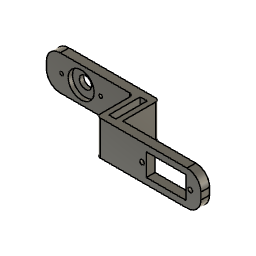
arm_2 v3 (Autodesk Fusion 360 design; units mm, degrees)
Autodesk Fusion 360 part; units mm, degrees
sketch "스케치1" plane through (0, 0, 0) normal (0, 0, 1) x (1, 0, 0)
sketch "스케치2" plane through (0, 0, 0) normal (0, 0, 1) x (1, 0, 0)
sketch "스케치3" plane through (0, 0, 0) normal (0, 0, 1) x (1, 0, 0)
sketch "스케치4" plane through (0, 0, 0) normal (0, 0, 1) x (1, 0, 0)
  line L0 (10, 5) -> (50, 5)
  line L1 (50, 5) -> (50, 0)
  line L2 (50, 0) -> (-20, 0)
  line L3 (-20, 0) -> (-20, 5)
  line L4 (10, 5) -> (10, 22)
  line L5 (10, 22) -> (-20, 22)
  line L6 (-20, 17) -> (-20, 5)
  line L7 (-20, 22) -> (-60, 22)
  line L8 (-60, 22) -> (-60, 17)
  line L9 (-60, 17) -> (-20, 17)
  constraint horizontal L0
  constraint vertical L1
  constraint horizontal L2
  constraint vertical L3
  constraint vertical L4
  constraint horizontal L5
  constraint vertical L6
  constraint horizontal L7
  constraint vertical L8
  constraint horizontal L9
extrude "돌출1" add sketch "스케치4" along normal blind 30
sketch "스케치5" plane through (0, 17, 0) normal (0, -1, 0) x (1, 0, 0)
  circle A0 centre (-40, 15) radius 3.5
  dimension "d3" = 7
  measures "d3" diameter of A0
hole "구멍1" at (-40, 17, 15) direction (0, 1, 0) diameter 7 depth 7 tip angle 118
sketch "스케치6" plane through (0, 17, 0) normal (0, -1, 0) x (1, 0, 0)
  circle A0 centre (-40, 15) radius 7.5
  dimension "d7" = 15
  measures "d7" diameter of A0
extrude "돌출2" cut sketch "스케치6" against normal blind 2.5
sketch "스케치7" plane through (0, 17, 0) normal (0, -1, 0) x (1, 0, 0)
  circle A0 centre (-51.25, 15) radius 1
  dimension "d10" = 2
  measures "d10" diameter of A0
hole "구멍2" at (-51.25, 17, 15) direction (0, 1, 0) diameter 2 depth 7 tip angle 118
sketch "스케치8" plane through (0, 17, 0) normal (0, -1, 0) x (1, 0, 0)
  circle A0 centre (-28.75, 15) radius 1
  dimension "d14" = 2
  measures "d14" diameter of A0
hole "구멍3" at (-28.75, 17, 15) direction (0, 1, 0) diameter 2 depth 7 tip angle 118
sketch "스케치9" plane through (0, 22, 0) normal (0, 1, 0) x (-1, 0, 0)
  circle A0 centre (51.25, 15) radius 1
  circle A1 centre (51.25, 15) radius 3.5
  circle A2 centre (28.75, 15) radius 1
  circle A3 centre (28.75, 15) radius 3.5
  dimension "d18" = 2
  dimension "d19" = 7
  dimension "d20" = 2
  dimension "d21" = 7
  constraint concentric A0 A1
  constraint concentric A2 A3
  measures "d18" diameter of A0
  measures "d19" diameter of A1
  measures "d20" diameter of A2
  measures "d21" diameter of A3
extrude "돌출3" cut sketch "스케치9" against normal blind 1 contours A1
sketch "스케치10" plane through (0, 22, 0) normal (0, 1, 0) x (-1, 0, 0)
  circle A0 centre (28.75, 15) radius 1
  circle A1 centre (28.75, 15) radius 3.5
  dimension "d24" = 2
  dimension "d25" = 7
  constraint concentric A0 A1
  measures "d24" diameter of A0
  measures "d25" diameter of A1
extrude "돌출4" cut sketch "스케치10" against normal blind 1
sketch "스케치11" plane through (0, 5, 0) normal (0, 1, 0) x (-1, 0, 0)
  line L0 (-18.6, 8.6) -> (-41.4, 8.6)
  line L1 (-41.4, 8.6) -> (-41.4, 21.4)
  line L2 (-41.4, 21.4) -> (-18.6, 21.4)
  line L3 (-18.6, 21.4) -> (-18.6, 8.6)
  line L4 (-18.6, 8.6) -> (-41.4, 21.4) construction
  line L5 (-41.4, 8.6) -> (-18.6, 21.4) construction
  point P0 (-30, 15)
  dimension "d28" = 22.8
  dimension "d29" = 12.8
  constraint horizontal L0
  constraint perpendicular L0 L1
  constraint parallel L0 L2
  constraint parallel L1 L3
  constraint coincident L4 P0
  constraint coincident L5 P0
  measures "d28" distance of L1.end L2.end
  measures "d29" distance of L0.end L1.end
extrude "돌출5" cut sketch "스케치11" against normal blind 5
sketch "스케치12" plane through (0, 5, 0) normal (0, 1, 0) x (-1, 0, 0)
  circle A0 centre (-43.9, 15) radius 1.3
  dimension "d32" = 2.6
  measures "d32" diameter of A0
extrude "돌출6" cut sketch "스케치12" against normal blind 5
sketch "스케치13" plane through (0, 5, 0) normal (0, 1, 0) x (-1, 0, 0)
  circle A0 centre (-16.1, 15) radius 1.3
  dimension "d35" = 2.6
  measures "d35" diameter of A0
extrude "돌출7" cut sketch "스케치13" against normal blind 5
extrude "돌출9" cut 1 faces at (-10, 7.3333, 30) along direction (0, 0, -1) blind 5
extrude "돌출10" cut 1 faces at (-10, 7.3333, 0) along direction (0, 0, 1) blind 5
extrude "돌출11" cut 1 faces at (10, 10.6667, 11.6667) along direction (-1, 0, 0) blind 10
extrude "돌출12" cut 1 faces at (-20, 5.6667, 11.6667) along direction (1, 0, 0) blind 10
move_face "면 이동1" to x (1, 0, 0) y (0, 1, 0) z (0, 0, 1) at (0, 4, 0) 12 faces at (-39.6515, 20.3333, 11.5174) (-31.4027, 21, 14.8012) (-28.6504, 18.3333, 14.005) (-53.9027, 21, 14.8012) (-15.9176, 17, 14.9751) (-33.8645, 19.5, 14.5402) (-51.7714, 18.3333, 15.8533) (-54.7326, 21.6667, 14.6515) (-60, 20.3333, 18.3333) (-8.4167, 22, 15) (-32.5093, 18.6667, 14.6262) (-32.2326, 21.6667, 14.6515)
fillet "모깎기18" radius 8 1 edges at (-60, 23.5, 25)
fillet "모깎기19" radius 2 1 edges at (-10, 21, 15)
fillet "모깎기20" radius 2 1 edges at (-10, 0, 15)
fillet "모깎기21" radius 8 1 edges at (-60, 23.5, 5)
fillet "모깎기22" radius 8 1 edges at (50, 2.5, 25)
fillet "모깎기23" radius 8 1 edges at (50, 2.5, 5)
fillet "모깎기24" radius 2 1 edges at (0, 26, 15)
sketch "스케치16" plane through (0, 0, 25) normal (0, 0, 1) x (-1, 0, 0)
  line L0 (7, -22) -> (3, -22)
  line L1 (3, -22) -> (3, -4)
  line L2 (3, -4) -> (7, -4)
  line L3 (7, -4) -> (7, -22)
  constraint horizontal L0
  constraint vertical L1
  constraint horizontal L2
  constraint vertical L3
extrude "돌출13" cut sketch "스케치16" against normal blind 20
sketch "스케치17" plane through (0, 26, 0) normal (0, 1, 0) x (-1, 0, 0)
fillet "모깎기10" [suppressed]
fillet "모깎기11" [suppressed]
fillet "모깎기12" [suppressed]
fillet "모깎기13" [suppressed]
fillet "모깎기14" [suppressed]
fillet "모깎기15" [suppressed]
fillet "모깎기16" [suppressed]
fillet "모깎기17" [suppressed]
sketch "스케치15" plane through (0, 0, 5) normal (0, 0, -1) x (1, 0, 0)
  line L0 (-7, -17) -> (-3, -17)
  line L1 (-3, -17) -> (-3, -3)
  line L2 (-3, -3) -> (-7, -3)
  line L3 (-7, -3) -> (-7, -17)
  line L4 (-7, -17) -> (-3, -3) construction
  line L5 (-3, -17) -> (-7, -3) construction
  point P0 (-5, -10)
  constraint horizontal L0
  constraint perpendicular L0 L1
  constraint parallel L0 L2
  constraint parallel L1 L3
  constraint coincident L4 P0
  constraint coincident L5 P0
fillet "모깎기1" [suppressed]
fillet "모깎기2" [suppressed]
fillet "모깎기3" [suppressed]
fillet "모깎기4" [suppressed]
fillet "모깎기5" [suppressed]
fillet "모깎기6" [suppressed]
fillet "모깎기7" [suppressed]
fillet "모깎기8" [suppressed]
fillet "모깎기9" [suppressed]
sketch "스케치14" plane through (0, 0, 0) normal (0, -1, 0) x (1, 0, 0)
  line L0 (5, 5) -> (-15, 5)
  line L1 (-15, 5) -> (-15, 25)
  line L2 (-15, 25) -> (5, 25)
  line L3 (5, 25) -> (5, 5)
  line L4 (5, 5) -> (-15, 25) construction
  line L5 (-15, 5) -> (5, 25) construction
  point P0 (-5, 15)
  constraint horizontal L0
  constraint perpendicular L0 L1
  constraint parallel L0 L2
  constraint parallel L1 L3
  constraint coincident L4 P0
  constraint coincident L5 P0
extrude "돌출8" [suppressed]
